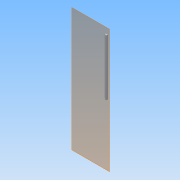
# Autodesk Inventor part: SideborderInverse
Saved by Autodesk Inventor 2013 (Build 170138000, 138)
## iProperties
Created: 2018-07-18
Part Number: SideborderInverse
Material: Generic
Document SubType Name: Modeling
Designer: Jeff Vyduna
Density: 1 g/cm^3
Author: Jeff Vyduna
Autodesk Inventor part; units mm, degrees
ref_plane "YZ Plane" through (0, 0, 0) normal (1, 0, 0) x (0, 1, 0)
ref_plane "XZ Plane" through (0, 0, 0) normal (0, 1, 0) x (-1, 0, 0)
ref_plane "XY Plane" through (0, 0, 0) normal (0, 0, 1) x (1, 0, 0)
ref_plane "Work Plane1" through (0, 0, 0) normal (0, 0, 1) x (1, 0, 0)
sketch "Sketch1" plane through (0, 0, 0) normal (0, 0, 1) x (1, 0, 0)
  line L0 (302.4187, 990.6) -> (264.3187, 990.6)
  line L1 (264.3187, 990.6) -> (264.3188, 0)
  line L2 (264.3188, 0) -> (302.4188, 0)
  line L3 (302.4188, 0) -> (302.4187, 990.6)
  point P0 (0, 0)
  dimension "d0" = 990.6
  dimension "d2" = 38.1
  constraints: 8 end point, 2 parallel, 1 coincident, 1 horizontal, 1 perpendicular, 1 other
  measures "d0" distance of L2.end L0.start
  measures "d2" distance of L0.start L0.end
extrude "Extrusion1" add sketch "Sketch1" along normal blind 25.4
sketch "Sketch3" plane through (0, 0, 25.4) normal (0, 0, 1) x (1, 0, 0)
  line L0 (264.3187, 990.6) -> (277.0187, 990.6)
  line L1 (277.0187, 990.6) -> (277.0187, 12.7)
  line L2 (277.0187, 12.7) -> (264.3187, 12.7)
  line L3 (264.3187, 12.7) -> (264.3187, 990.6)
  point P0 (0, 0)
  dimension "d10" = 12.7
  dimension "d11" = 977.9
  constraints: 8 end point, 2 parallel, 1 horizontal, 1 perpendicular
  measures "d10" distance of L1.end L2.end
  measures "d11" distance of L0.end L1.end
extrude "Extrusion3" cut sketch "Sketch3" against normal blind 8.4646
equation "\"d0\" = 0.5 * signH"
equation "\"d2\" = borderW"
equation "\"d3\" = borderH"
equation "\"d10\" = panelLap"
equation "\"d11\" = 0.5 * signH - panelLap"
equation "\"d12\" = panelH + velcroH + panelHClear"
equation "\"signH\" = 1981.2"
equation "\"borderW\" = 38.1"
equation "\"borderH\" = 25.4"
equation "\"velcroH\" = 2.54"
equation "\"panelH\" = 5.1308"
equation "\"panelHClear\" = 0.79375"
equation "\"panelLap\" = 12.7"
body "Solid1"
